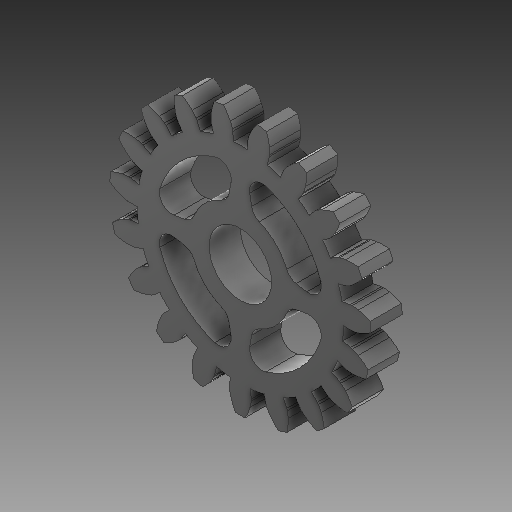
# Autodesk Inventor part: 歯車m2.z19
Saved by Autodesk Inventor 2020 (Build 240168000, 168)
## iProperties
Created: 2019-07-07
Part Number: 歯車m2.z19
Material: アセタール樹脂、黒
Document SubType Name: Modeling
Designer: 雪村
Density: 1.425 g/cm^3
Appearance: 滑らか - 黒
Mass: 5.2471 g
Surface Area: 35.7031 cm^2
Volume: 3.68217 cm^3
Description: ジュラコン 5t
Author: 雪村
Autodesk Inventor part; units mm, degrees
ref_plane "YZ Plane" through (0, 0, 0) normal (1, 0, 0) x (0, 1, 0)
ref_plane "XZ Plane" through (0, 0, 0) normal (0, 1, 0) x (-1, 0, 0)
ref_plane "XY Plane" through (0, 0, 0) normal (0, 0, 1) x (1, 0, 0)
sketch "スケッチ1" plane through (0, 0, 0) normal (0, 0, 1) x (1, 0, 0)
  arc A0 (20.2426, 88.5604) -> (20.1852, 88.263) centre (22.0204, 88.0631) ccw
  arc A1 (20.595, 89.4907) -> (20.2426, 88.5604) centre (25.1554, 87.231) ccw
  arc A2 (21.6786, 91.1755) -> (20.595, 89.4907) centre (28.5313, 85.5773) ccw
  arc A3 (14.2935, 87.9903) -> (14.3357, 87.6904) centre (16.1364, 88.0972) ccw
  arc A4 (14.3247, 88.9847) -> (14.2935, 87.9903) centre (19.3717, 88.3282) ccw
  arc A5 (14.8026, 90.93) -> (14.3247, 88.9847) centre (23.1017, 87.8602) ccw
  arc A6 (8.8518, 85.5195) -> (8.9892, 85.2495) centre (10.5602, 86.2189) ccw
  arc A7 (8.5585, 86.4701) -> (8.8518, 85.5195) centre (13.5452, 87.4879) ccw
  arc A8 (8.3788, 88.4651) -> (8.5585, 86.4701) centre (17.225, 88.2564) ccw
  arc A9 (4.5072, 81.4156) -> (4.7248, 81.2048) centre (5.8959, 82.6319) ccw
  arc A10 (3.9212, 82.2195) -> (4.5072, 81.4156) centre (8.3072, 84.8013) ccw
  arc A11 (3.1034, 84.0481) -> (3.9212, 82.2195) centre (11.5381, 86.723) ccw
  arc A12 (1.7306, 76.1234) -> (2.0048, 75.9947) centre (2.6491, 77.7247) ccw
  arc A13 (0.9153, 76.6934) -> (1.7306, 76.1234) centre (4.2253, 80.5595) ccw
  arc A14 (-0.4519, 78.1574) -> (0.9153, 76.6934) centre (6.6572, 83.4261) ccw
  arc A15 (0.8228, 70.2163) -> (1.124, 70.1837) centre (1.1716, 72.0291) ccw
  arc A16 (-0.1334, 70.4908) -> (0.8228, 70.2163) centre (1.742, 75.2221) ccw
  arc A17 (-1.9019, 71.4315) -> (-0.1334, 70.4908) centre (3.1113, 78.7231) ccw
  arc A18 (1.8822, 64.3346) -> (2.1776, 64.4015) centre (1.6235, 66.1624) ccw
  arc A19 (0.8887, 64.2837) -> (1.8822, 64.3346) centre (1.1262, 69.3676) ccw
  arc A20 (-1.0894, 64.5992) -> (0.8887, 64.2837) centre (1.2845, 73.1235) ccw
  arc A21 (4.794, 59.1156) -> (5.0517, 59.2748) centre (3.9558, 60.7604) ccw
  arc A22 (3.8708, 58.7448) -> (4.794, 59.1156) centre (2.4447, 63.6304) ccw
  arc A23 (1.8975, 58.401) -> (3.8708, 58.7448) centre (1.375, 67.2342) ccw
  arc A24 (9.2427, 55.1248) -> (9.4347, 55.359) centre (7.9158, 56.4083) ccw
  arc A25 (8.4899, 54.4743) -> (9.2427, 55.1248) centre (5.5547, 58.6321) ccw
  arc A26 (6.7351, 53.5084) -> (8.4899, 54.4743) centre (3.3728, 61.6933) ccw
  arc A27 (14.7461, 52.7947) -> (14.8516, 53.0786) centre (13.0744, 53.5778) ccw
  arc A28 (14.2453, 51.9351) -> (14.7461, 52.7947) centre (10.1191, 54.9145) ccw
  arc A29 (12.8992, 50.4516) -> (14.2453, 51.9351) centre (7.0614, 57.1014) ccw
  arc A30 (20.7079, 52.3778) -> (20.7155, 52.6806) centre (18.8725, 52.5757) ccw
  arc A31 (20.5134, 51.4021) -> (20.7079, 52.3778) centre (15.6433, 52.8804) ccw
  arc A32 (19.7219, 49.562) -> (20.5134, 51.4021) centre (12.0412, 53.9559) ccw
  arc A33 (26.482, 53.9192) -> (26.391, 54.2081) centre (24.6818, 53.5105) ccw
  arc A34 (26.6148, 52.9333) -> (26.482, 53.9192) centre (21.5286, 52.7502) ccw
  arc A35 (26.4637, 50.9359) -> (26.6148, 52.9333) centre (17.7725, 52.5978) ccw
  arc A36 (31.4428, 57.2521) -> (31.2629, 57.4958) centre (29.8729, 56.281) ccw
  arc A37 (31.8885, 56.3627) -> (31.4428, 57.2521) centre (27.1374, 54.538) ccw
  arc A38 (32.3942, 54.4244) -> (31.8885, 56.3627) centre (23.6343, 53.1743) ccw
  arc A39 (35.0526, 62.0151) -> (34.8033, 62.1871) centre (33.8831, 60.5868) ccw
  arc A40 (35.763, 61.3186) -> (35.0526, 62.0151) centre (31.8618, 58.0501) ccw
  arc A41 (36.8706, 59.6496) -> (35.763, 61.3186) centre (28.9912, 55.6228) ccw
  arc A42 (36.9203, 67.6921) -> (36.6286, 67.7739) centre (36.2779, 65.9615) ccw
  arc A43 (37.8183, 67.2641) -> (36.9203, 67.6921) centre (35.1898, 62.9059) ccw
  arc A44 (39.4078, 66.0451) -> (37.8183, 67.2641) centre (33.2629, 59.6781) ccw
  arc A45 (36.8435, 73.668) -> (36.541, 73.6506) centre (36.7978, 71.8225) ccw
  arc A46 (37.8318, 73.5547) -> (36.8435, 73.668) centre (36.7608, 68.5792) ccw
  arc A47 (39.731, 72.9179) -> (37.8318, 73.5547) centre (35.9864, 64.9006) ccw
  arc A48 (34.8304, 79.2951) -> (34.55, 79.1805) centre (35.3864, 77.5348) ccw
  arc A49 (35.802, 79.5089) -> (34.8304, 79.2951) centre (36.4045, 74.4552) ccw
  arc A50 (37.8051, 79.5233) -> (35.802, 79.5089) centre (36.8665, 70.7245) ccw
  arc A51 (31.0993, 83.9638) -> (30.8713, 83.7643) centre (32.1968, 82.4793) ccw
  arc A52 (31.9488, 84.4814) -> (31.0993, 83.9638) centre (34.1597, 79.8972) ccw
  arc A53 (33.8387, 85.1454) -> (31.9488, 84.4814) centre (35.808, 76.5186) ccw
  arc A54 (26.0545, 87.1679) -> (25.9036, 86.9052) centre (27.5744, 86.1203) ccw
  arc A55 (26.6899, 87.9334) -> (26.0545, 87.1679) centre (30.2694, 84.3154) ccw
  arc A56 (28.2618, 89.175) -> (26.6899, 87.9334) centre (32.9254, 81.6551) ccw
  arc A57 (17.7671, 88.263) -> (17.7097, 88.5604) centre (15.9319, 88.0631) ccw
  arc A58 (17.7097, 88.5604) -> (17.3572, 89.4907) centre (12.7969, 87.231) ccw
  arc A59 (17.3572, 89.4907) -> (16.2737, 91.1755) centre (9.421, 85.5773) ccw
  arc A60 (12.0487, 86.9052) -> (11.8978, 87.1679) centre (10.3778, 86.1203) ccw
  arc A61 (11.8978, 87.1679) -> (11.2624, 87.9334) centre (7.6829, 84.3154) ccw
  arc A62 (11.2624, 87.9334) -> (9.6905, 89.175) centre (5.0268, 81.6551) ccw
  arc A63 (7.081, 83.7643) -> (6.853, 83.9638) centre (5.7555, 82.4793) ccw
  arc A64 (6.853, 83.9638) -> (6.0034, 84.4814) centre (3.7926, 79.8972) ccw
  arc A65 (6.0034, 84.4814) -> (4.1136, 85.1454) centre (2.1443, 76.5186) ccw
  arc A66 (3.4023, 79.1805) -> (3.1219, 79.2951) centre (2.5659, 77.5348) ccw
  arc A67 (3.1219, 79.2951) -> (2.1503, 79.5089) centre (1.5477, 74.4552) ccw
  arc A68 (2.1503, 79.5089) -> (0.1472, 79.5233) centre (1.0857, 70.7245) ccw
  arc A69 (1.4112, 73.6506) -> (1.1088, 73.668) centre (1.1545, 71.8225) ccw
  arc A70 (1.1088, 73.668) -> (0.1205, 73.5547) centre (1.1915, 68.5792) ccw
  arc A71 (0.1205, 73.5547) -> (-1.7787, 72.9179) centre (1.9659, 64.9006) ccw
  arc A72 (1.3236, 67.7739) -> (1.032, 67.6921) centre (1.6744, 65.9615) ccw
  arc A73 (1.032, 67.6921) -> (0.134, 67.2641) centre (2.7625, 62.9059) ccw
  arc A74 (0.134, 67.2641) -> (-1.4556, 66.0451) centre (4.6894, 59.6781) ccw
  arc A75 (3.149, 62.1871) -> (2.8997, 62.0151) centre (4.0692, 60.5868) ccw
  arc A76 (2.8997, 62.0151) -> (2.1893, 61.3186) centre (6.0905, 58.0501) ccw
  arc A77 (2.1893, 61.3186) -> (1.0817, 59.6496) centre (8.961, 55.6228) ccw
  arc A78 (6.6894, 57.4958) -> (6.5095, 57.2521) centre (8.0794, 56.281) ccw
  arc A79 (6.5095, 57.2521) -> (6.0637, 56.3627) centre (10.8149, 54.538) ccw
  arc A80 (6.0637, 56.3627) -> (5.5581, 54.4244) centre (14.318, 53.1743) ccw
  arc A81 (11.5613, 54.2081) -> (11.4702, 53.9192) centre (13.2705, 53.5105) ccw
  arc A82 (11.4702, 53.9192) -> (11.3374, 52.9333) centre (16.4236, 52.7502) ccw
  arc A83 (11.3374, 52.9333) -> (11.4886, 50.9359) centre (20.1797, 52.5978) ccw
  arc A84 (17.2367, 52.6806) -> (17.2444, 52.3778) centre (19.0798, 52.5757) ccw
  arc A85 (17.2444, 52.3778) -> (17.4389, 51.4021) centre (22.309, 52.8804) ccw
  arc A86 (17.4389, 51.4021) -> (18.2304, 49.562) centre (25.9111, 53.9559) ccw
  arc A87 (23.1006, 53.0786) -> (23.2062, 52.7947) centre (24.8779, 53.5778) ccw
  arc A88 (23.2062, 52.7947) -> (23.707, 51.9351) centre (27.8332, 54.9145) ccw
  arc A89 (23.707, 51.9351) -> (25.0531, 50.4516) centre (30.8909, 57.1014) ccw
  arc A90 (28.5176, 55.359) -> (28.7096, 55.1248) centre (30.0364, 56.4083) ccw
  arc A91 (28.7096, 55.1248) -> (29.4624, 54.4743) centre (32.3976, 58.6321) ccw
  arc A92 (29.4624, 54.4743) -> (31.2172, 53.5084) centre (34.5795, 61.6933) ccw
  arc A93 (32.9006, 59.2748) -> (33.1583, 59.1156) centre (33.9964, 60.7604) ccw
  arc A94 (33.1583, 59.1156) -> (34.0814, 58.7448) centre (35.5076, 63.6304) ccw
  arc A95 (34.0814, 58.7448) -> (36.0548, 58.401) centre (36.5773, 67.2342) ccw
  arc A96 (35.7746, 64.4015) -> (36.0701, 64.3346) centre (36.3288, 66.1624) ccw
  arc A97 (36.0701, 64.3346) -> (37.0636, 64.2837) centre (36.8261, 69.3676) ccw
  arc A98 (37.0636, 64.2837) -> (39.0417, 64.5992) centre (36.6678, 73.1235) ccw
  arc A99 (36.8283, 70.1837) -> (37.1295, 70.2163) centre (36.7806, 72.0291) ccw
  arc A100 (37.1295, 70.2163) -> (38.0857, 70.4908) centre (36.2103, 75.2221) ccw
  arc A101 (38.0857, 70.4908) -> (39.8542, 71.4315) centre (34.841, 78.7231) ccw
  arc A102 (35.9474, 75.9947) -> (36.2217, 76.1234) centre (35.3031, 77.7247) ccw
  arc A103 (36.2217, 76.1234) -> (37.037, 76.6934) centre (33.727, 80.5595) ccw
  arc A104 (37.037, 76.6934) -> (38.4042, 78.1574) centre (31.2951, 83.4261) ccw
  arc A105 (33.2275, 81.2048) -> (33.4451, 81.4156) centre (32.0563, 82.6319) ccw
  arc A106 (33.4451, 81.4156) -> (34.0311, 82.2195) centre (29.6451, 84.8013) ccw
  arc A107 (34.0311, 82.2195) -> (34.8489, 84.0481) centre (26.4142, 86.723) ccw
  arc A108 (28.9631, 85.2495) -> (29.1005, 85.5195) centre (27.3921, 86.2189) ccw
  arc A109 (29.1005, 85.5195) -> (29.3938, 86.4701) centre (24.4071, 87.4879) ccw
  arc A110 (29.3938, 86.4701) -> (29.5735, 88.4651) centre (20.7273, 88.2564) ccw
  arc A111 (23.6165, 87.6904) -> (23.6588, 87.9903) centre (21.8159, 88.0972) ccw
  arc A112 (23.6588, 87.9903) -> (23.6275, 88.9847) centre (18.5806, 88.3282) ccw
  arc A113 (23.6275, 88.9847) -> (23.1497, 90.93) centre (14.8506, 87.8602) ccw
  arc A114 (20.0935, 86.9119) -> (17.8588, 86.9119) centre (18.9761, 70.4498) ccw
  arc A115 (14.6877, 86.3828) -> (12.5741, 85.6572) centre (18.9761, 70.4498) ccw
  arc A116 (9.7466, 84.127) -> (7.9832, 82.7545) centre (18.9761, 70.4498) ccw
  arc A117 (5.8057, 80.3891) -> (4.5835, 78.5183) centre (18.9761, 70.4498) ccw
  arc A118 (3.292, 75.5742) -> (2.7435, 73.4079) centre (18.9761, 70.4498) ccw
  arc A119 (2.478, 70.2039) -> (2.6625, 67.9769) centre (18.9761, 70.4498) ccw
  arc A120 (3.4517, 64.8603) -> (4.3494, 62.8138) centre (18.9761, 70.4498) ccw
  arc A121 (6.1078, 60.1224) -> (7.6213, 58.4783) centre (18.9761, 70.4498) ccw
  arc A122 (10.1584, 56.5036) -> (12.1237, 55.44) centre (18.9761, 70.4498) ccw
  arc A123 (15.1645, 54.3961) -> (17.3687, 54.0283) centre (18.9761, 70.4498) ccw
  arc A124 (20.5836, 54.0283) -> (22.7878, 54.3961) centre (18.9761, 70.4498) ccw
  arc A125 (25.8286, 55.44) -> (27.7939, 56.5036) centre (18.9761, 70.4498) ccw
  arc A126 (30.331, 58.4783) -> (31.8445, 60.1224) centre (18.9761, 70.4498) ccw
  arc A127 (33.6029, 62.8138) -> (34.5005, 64.8603) centre (18.9761, 70.4498) ccw
  arc A128 (35.2898, 67.9769) -> (35.4743, 70.2039) centre (18.9761, 70.4498) ccw
  arc A129 (35.2088, 73.4079) -> (34.6602, 75.5742) centre (18.9761, 70.4498) ccw
  arc A130 (33.3688, 78.5183) -> (32.1466, 80.3891) centre (18.9761, 70.4498) ccw
  arc A131 (29.9691, 82.7545) -> (28.2057, 84.127) centre (18.9761, 70.4498) ccw
  arc A132 (25.3782, 85.6572) -> (23.2646, 86.3828) centre (18.9761, 70.4498) ccw
  arc A133 (16.2737, 91.1755) -> (14.8026, 90.93) centre (18.9761, 70.4498) ccw
  arc A134 (9.6905, 89.175) -> (8.3788, 88.4651) centre (18.9761, 70.4498) ccw
  arc A135 (4.1136, 85.1454) -> (3.1034, 84.0481) centre (18.9761, 70.4498) ccw
  arc A136 (0.1472, 79.5233) -> (-0.4519, 78.1574) centre (18.9761, 70.4498) ccw
  arc A137 (-1.7787, 72.9179) -> (-1.9019, 71.4315) centre (18.9761, 70.4498) ccw
  arc A138 (-1.4556, 66.0451) -> (-1.0894, 64.5992) centre (18.9761, 70.4498) ccw
  arc A139 (1.0817, 59.6496) -> (1.8975, 58.401) centre (18.9761, 70.4498) ccw
  arc A140 (5.5581, 54.4244) -> (6.7351, 53.5084) centre (18.9761, 70.4498) ccw
  arc A141 (11.4886, 50.9359) -> (12.8992, 50.4516) centre (18.9761, 70.4498) ccw
  arc A142 (18.2304, 49.562) -> (19.7219, 49.562) centre (18.9761, 70.4498) ccw
  arc A143 (25.0531, 50.4516) -> (26.4637, 50.9359) centre (18.9761, 70.4498) ccw
  arc A144 (31.2172, 53.5084) -> (32.3942, 54.4244) centre (18.9761, 70.4498) ccw
  arc A145 (36.0548, 58.401) -> (36.8706, 59.6496) centre (18.9761, 70.4498) ccw
  arc A146 (39.0417, 64.5992) -> (39.4078, 66.0451) centre (18.9761, 70.4498) ccw
  arc A147 (39.8542, 71.4315) -> (39.731, 72.9179) centre (18.9761, 70.4498) ccw
  arc A148 (38.4042, 78.1574) -> (37.8051, 79.5233) centre (18.9761, 70.4498) ccw
  arc A149 (34.8489, 84.0481) -> (33.8387, 85.1454) centre (18.9761, 70.4498) ccw
  arc A150 (29.5735, 88.4651) -> (28.2618, 89.175) centre (18.9761, 70.4498) ccw
  arc A151 (23.1497, 90.93) -> (21.6786, 91.1755) centre (18.9761, 70.4498) ccw
  line L0 (20.0935, 86.9119) -> (20.1852, 88.263)
  line L1 (14.6877, 86.3828) -> (14.3357, 87.6904)
  line L2 (9.7466, 84.127) -> (8.9892, 85.2495)
  line L3 (5.8057, 80.3891) -> (4.7248, 81.2048)
  line L4 (3.292, 75.5742) -> (2.0048, 75.9947)
  line L5 (2.478, 70.2039) -> (1.124, 70.1837)
  line L6 (3.4517, 64.8603) -> (2.1776, 64.4015)
  line L7 (6.1078, 60.1224) -> (5.0517, 59.2748)
  line L8 (10.1584, 56.5036) -> (9.4347, 55.359)
  line L9 (15.1645, 54.3961) -> (14.8516, 53.0786)
  line L10 (20.5836, 54.0283) -> (20.7155, 52.6806)
  line L11 (25.8286, 55.44) -> (26.391, 54.2081)
  line L12 (30.331, 58.4783) -> (31.2629, 57.4958)
  line L13 (33.6029, 62.8138) -> (34.8033, 62.1871)
  line L14 (35.2898, 67.9769) -> (36.6286, 67.7739)
  line L15 (35.2088, 73.4079) -> (36.541, 73.6506)
  line L16 (33.3688, 78.5183) -> (34.55, 79.1805)
  line L17 (29.9691, 82.7545) -> (30.8713, 83.7643)
  line L18 (25.3782, 85.6572) -> (25.9036, 86.9052)
  line L19 (17.8588, 86.9119) -> (17.7671, 88.263)
  line L20 (12.5741, 85.6572) -> (12.0487, 86.9052)
  line L21 (7.9832, 82.7545) -> (7.081, 83.7643)
  line L22 (4.5835, 78.5183) -> (3.4023, 79.1805)
  line L23 (2.7435, 73.4079) -> (1.4112, 73.6506)
  line L24 (2.6625, 67.9769) -> (1.3236, 67.7739)
  line L25 (4.3494, 62.8138) -> (3.149, 62.1871)
  line L26 (7.6213, 58.4783) -> (6.6894, 57.4958)
  line L27 (12.1237, 55.44) -> (11.5613, 54.2081)
  line L28 (17.3687, 54.0283) -> (17.2367, 52.6806)
  line L29 (22.7878, 54.3961) -> (23.1006, 53.0786)
  line L30 (27.7939, 56.5036) -> (28.5176, 55.359)
  line L31 (31.8445, 60.1224) -> (32.9006, 59.2748)
  line L32 (34.5005, 64.8603) -> (35.7746, 64.4015)
  line L33 (35.4743, 70.2039) -> (36.8283, 70.1837)
  line L34 (34.6602, 75.5742) -> (35.9474, 75.9947)
  line L35 (32.1466, 80.3891) -> (33.2275, 81.2048)
  line L36 (28.2057, 84.127) -> (28.9631, 85.2495)
  line L37 (23.2646, 86.3828) -> (23.6165, 87.6904)
  line L38 (-3.925, 70.4498) -> (41.8772, 70.4498)
  line L39 (18.9761, 47.5487) -> (18.9761, 93.3509)
  line L40 (59.8772, 91.3509) -> (129.8772, 91.3509)
  line L41 (59.8772, 83.3509) -> (129.8772, 83.3509)
  line L42 (59.8772, 75.3509) -> (129.8772, 75.3509)
  line L43 (59.8772, 67.3509) -> (129.8772, 67.3509)
  line L44 (59.8772, 59.3509) -> (129.8772, 59.3509)
  line L45 (59.8772, 51.3509) -> (129.8772, 51.3509)
  line L46 (59.8772, 43.3509) -> (129.8772, 43.3509)
  line L47 (59.8772, 35.3509) -> (129.8772, 35.3509)
  line L48 (59.8772, 27.3509) -> (129.8772, 27.3509)
  line L49 (59.8772, 19.3509) -> (129.8772, 19.3509)
  line L50 (59.8772, 11.3509) -> (129.8772, 11.3509)
  line L51 (59.8772, 3.3509) -> (129.8772, 3.3509)
  line L52 (59.8772, -4.6491) -> (129.8772, -4.6491)
  line L53 (59.8772, 91.3509) -> (59.8772, -4.6491)
  line L54 (129.8772, 91.3509) -> (129.8772, -4.6491)
  line L55 (94.8772, 83.3509) -> (94.8772, -4.6491)
  point P0 (0, 0)
  point P1 (0, 0)
  point P2 (65.8772, 85.3509)
  point P3 (68.3772, 77.3509)
  point P4 (68.3772, 69.3509)
  point P5 (65.8772, 61.3509)
  point P6 (68.3772, 53.3509)
  point P7 (63.3772, 45.3509)
  point P8 (65.8772, 37.3509)
  point P9 (65.8772, 29.3509)
  point P10 (65.8772, 21.3509)
  point P11 (68.3772, 13.3509)
  point P12 (68.3772, 5.3509)
  point P13 (65.8772, -2.6491)
  point P14 (95.8772, 77.3509)
  point P15 (110.8772, 69.3509)
  point P16 (112.1272, 61.3509)
  point P17 (108.3772, 53.3509)
  point P18 (110.8772, 45.3509)
  point P19 (104.6272, 37.3509)
  point P20 (104.6272, 29.3509)
  point P21 (110.8772, 21.3509)
  point P22 (105.8772, 13.3509)
  point P23 (19.9761, 106.8509)
  point P24 (19.9761, 100.8509)
  point P25 (36.1636, 106.8509)
  point P26 (39.3511, 100.8509)
  constraints: 228 point on circle, 114 centre point, 108 end point, 2 horizontal alignment, 2 midpoint, 165 other
extrude "押し出し1" add sketch "スケッチ1" along normal blind 5 contours A1 A2 A151 A113 A112 A111 L37 A132 L18 A54 A55 A56 A150 A110 A109 A108 L36 A131 L17 A51 A52 A53 A149 A107 A106 A105 L35 A130 L16 A48 A49 A50 A148 A104 A103 A102 L34 A129 L15 A45 A46 A47 A147 A101 A100 L38 L39 A114 L0 A0 | L39 L38 A16 A17 A137 A71 A70 A69 L23 A118 L4 A12 A13 A14 A136 A68 A67 A66 L22 A117 L3 A9 A10 A11 A135 A65 A64 A63 L21 A116 L2 A6 A7 A8 A134 A62 A61 A60 L20 A115 L1 A3 A4 A5 A133 A59 A58 A57 L19 A114 | L39 A142 A86 A85 A84 L28 A123 L9 A27 A28 A29 A141 A83 A82 A81 L27 A122 L8 A24 A25 A26 A140 A80 A79 A78 L26 A121 L7 A21 A22 A23 A139 A77 A76 A75 L25 A120 L6 A18 A19 A20 A138 A74 A73 A72 L24 A119 L5 A15 A16 L38 | L38 A100 A99 L33 A128 L14 A42 A43 A44 A146 A98 A97 A96 L32 A127 L13 A39 A40 A41 A145 A95 A94 A93 L31 A126 L12 A36 A37 A38 A144 A92 A91 A90 L30 A125 L11 A33 A34 A35 A143 A89 A88 A87 L29 A124 L10 A30 A31 A32 A142 L39
sketch "スケッチ2" plane through (0, 0, 5) normal (0, 0, 1) x (1, 0, 0)
  arc A0 (6.5095, 57.2521) -> (6.0637, 56.3627) centre (10.8149, 54.538) ccw projected
  arc A1 (6.0637, 56.3627) -> (5.5581, 54.4244) centre (14.318, 53.1743) ccw projected
  arc A2 (5.5581, 54.4244) -> (6.7351, 53.5084) centre (18.9761, 70.4498) ccw projected
  arc A3 (6.7351, 53.5084) -> (8.4899, 54.4743) centre (3.3728, 61.6933) ccw projected
  arc A4 (8.4899, 54.4743) -> (9.2427, 55.1248) centre (5.5547, 58.6321) ccw projected
  arc A5 (9.2427, 55.1248) -> (9.4347, 55.359) centre (7.9158, 56.4083) ccw projected
  line L0 (9.4347, 55.359) -> (10.1584, 56.5036) projected
  arc A6 (10.1584, 56.5036) -> (12.1237, 55.44) centre (18.9761, 70.4498) ccw projected
  line L1 (12.1237, 55.44) -> (11.5613, 54.2081) projected
  arc A7 (11.5613, 54.2081) -> (11.4702, 53.9192) centre (13.2705, 53.5105) ccw projected
  arc A8 (11.4702, 53.9192) -> (11.3374, 52.9333) centre (16.4236, 52.7502) ccw projected
  arc A9 (11.3374, 52.9333) -> (11.4886, 50.9359) centre (20.1797, 52.5978) ccw projected
  arc A10 (11.4886, 50.9359) -> (12.8992, 50.4516) centre (18.9761, 70.4498) ccw projected
  arc A11 (12.8992, 50.4516) -> (14.2453, 51.9351) centre (7.0614, 57.1014) ccw projected
  arc A12 (14.2453, 51.9351) -> (14.7461, 52.7947) centre (10.1191, 54.9145) ccw projected
  arc A13 (14.7461, 52.7947) -> (14.8516, 53.0786) centre (13.0744, 53.5778) ccw projected
  line L2 (14.8516, 53.0786) -> (15.1645, 54.3961) projected
  arc A14 (15.1645, 54.3961) -> (17.3687, 54.0283) centre (18.9761, 70.4498) ccw projected
  line L3 (17.3687, 54.0283) -> (17.2367, 52.6806) projected
  arc A15 (17.2367, 52.6806) -> (17.2444, 52.3778) centre (19.0798, 52.5757) ccw projected
  arc A16 (17.2444, 52.3778) -> (17.4389, 51.4021) centre (22.309, 52.8804) ccw projected
  arc A17 (17.4389, 51.4021) -> (18.2304, 49.562) centre (25.9111, 53.9559) ccw projected
  arc A18 (18.2304, 49.562) -> (19.7219, 49.562) centre (18.9761, 70.4498) ccw projected
  arc A19 (19.7219, 49.562) -> (20.5134, 51.4021) centre (12.0412, 53.9559) ccw projected
  arc A20 (20.5134, 51.4021) -> (20.7079, 52.3778) centre (15.6433, 52.8804) ccw projected
  arc A21 (20.7079, 52.3778) -> (20.7155, 52.6806) centre (18.8725, 52.5757) ccw projected
  line L4 (20.7155, 52.6806) -> (20.5836, 54.0283) projected
  arc A22 (20.5836, 54.0283) -> (22.7878, 54.3961) centre (18.9761, 70.4498) ccw projected
  line L5 (22.7878, 54.3961) -> (23.1006, 53.0786) projected
  arc A23 (23.1006, 53.0786) -> (23.2062, 52.7947) centre (24.8779, 53.5778) ccw projected
  arc A24 (23.2062, 52.7947) -> (23.707, 51.9351) centre (27.8332, 54.9145) ccw projected
  arc A25 (23.707, 51.9351) -> (25.0531, 50.4516) centre (30.8909, 57.1014) ccw projected
  arc A26 (25.0531, 50.4516) -> (26.4637, 50.9359) centre (18.9761, 70.4498) ccw projected
  arc A27 (26.4637, 50.9359) -> (26.6148, 52.9333) centre (17.7725, 52.5978) ccw projected
  arc A28 (26.6148, 52.9333) -> (26.482, 53.9192) centre (21.5286, 52.7502) ccw projected
  arc A29 (26.482, 53.9192) -> (26.391, 54.2081) centre (24.6818, 53.5105) ccw projected
  line L6 (26.391, 54.2081) -> (25.8286, 55.44) projected
  arc A30 (25.8286, 55.44) -> (27.7939, 56.5036) centre (18.9761, 70.4498) ccw projected
  line L7 (27.7939, 56.5036) -> (28.5176, 55.359) projected
  arc A31 (28.5176, 55.359) -> (28.7096, 55.1248) centre (30.0364, 56.4083) ccw projected
  arc A32 (28.7096, 55.1248) -> (29.4624, 54.4743) centre (32.3976, 58.6321) ccw projected
  arc A33 (29.4624, 54.4743) -> (31.2172, 53.5084) centre (34.5795, 61.6933) ccw projected
  arc A34 (31.2172, 53.5084) -> (32.3942, 54.4244) centre (18.9761, 70.4498) ccw projected
  arc A35 (32.3942, 54.4244) -> (31.8885, 56.3627) centre (23.6343, 53.1743) ccw projected
  arc A36 (31.8885, 56.3627) -> (31.4428, 57.2521) centre (27.1374, 54.538) ccw projected
  arc A37 (31.4428, 57.2521) -> (31.2629, 57.4958) centre (29.8729, 56.281) ccw projected
  line L8 (31.2629, 57.4958) -> (30.331, 58.4783) projected
  arc A38 (30.331, 58.4783) -> (31.8445, 60.1224) centre (18.9761, 70.4498) ccw projected
  line L9 (31.8445, 60.1224) -> (32.9006, 59.2748) projected
  arc A39 (32.9006, 59.2748) -> (33.1583, 59.1156) centre (33.9964, 60.7604) ccw projected
  arc A40 (33.1583, 59.1156) -> (34.0814, 58.7448) centre (35.5076, 63.6304) ccw projected
  arc A41 (34.0814, 58.7448) -> (36.0548, 58.401) centre (36.5773, 67.2342) ccw projected
  arc A42 (36.0548, 58.401) -> (36.8706, 59.6496) centre (18.9761, 70.4498) ccw projected
  arc A43 (36.8706, 59.6496) -> (35.763, 61.3186) centre (28.9912, 55.6228) ccw projected
  arc A44 (35.763, 61.3186) -> (35.0526, 62.0151) centre (31.8618, 58.0501) ccw projected
  arc A45 (35.0526, 62.0151) -> (34.8033, 62.1871) centre (33.8831, 60.5868) ccw projected
  line L10 (34.8033, 62.1871) -> (33.6029, 62.8138) projected
  arc A46 (33.6029, 62.8138) -> (34.5005, 64.8603) centre (18.9761, 70.4498) ccw projected
  line L11 (34.5005, 64.8603) -> (35.7746, 64.4015) projected
  arc A47 (35.7746, 64.4015) -> (36.0701, 64.3346) centre (36.3288, 66.1624) ccw projected
  arc A48 (36.0701, 64.3346) -> (37.0636, 64.2837) centre (36.8261, 69.3676) ccw projected
  arc A49 (37.0636, 64.2837) -> (39.0417, 64.5992) centre (36.6678, 73.1235) ccw projected
  arc A50 (39.0417, 64.5992) -> (39.4078, 66.0451) centre (18.9761, 70.4498) ccw projected
  arc A51 (39.4078, 66.0451) -> (37.8183, 67.2641) centre (33.2629, 59.6781) ccw projected
  arc A52 (37.8183, 67.2641) -> (36.9203, 67.6921) centre (35.1898, 62.9059) ccw projected
  arc A53 (36.9203, 67.6921) -> (36.6286, 67.7739) centre (36.2779, 65.9615) ccw projected
  line L12 (36.6286, 67.7739) -> (35.2898, 67.9769) projected
  arc A54 (35.2898, 67.9769) -> (35.4743, 70.2039) centre (18.9761, 70.4498) ccw projected
  line L13 (35.4743, 70.2039) -> (36.8283, 70.1837) projected
  arc A55 (36.8283, 70.1837) -> (37.1295, 70.2163) centre (36.7806, 72.0291) ccw projected
  arc A56 (37.1295, 70.2163) -> (38.0857, 70.4908) centre (36.2103, 75.2221) ccw projected
  arc A57 (38.0857, 70.4908) -> (39.8542, 71.4315) centre (34.841, 78.7231) ccw projected
  arc A58 (39.8542, 71.4315) -> (39.731, 72.9179) centre (18.9761, 70.4498) ccw projected
  arc A59 (39.731, 72.9179) -> (37.8318, 73.5547) centre (35.9864, 64.9006) ccw projected
  arc A60 (37.8318, 73.5547) -> (36.8435, 73.668) centre (36.7608, 68.5792) ccw projected
  arc A61 (36.8435, 73.668) -> (36.541, 73.6506) centre (36.7978, 71.8225) ccw projected
  line L14 (36.541, 73.6506) -> (35.2088, 73.4079) projected
  arc A62 (35.2088, 73.4079) -> (34.6602, 75.5742) centre (18.9761, 70.4498) ccw projected
  line L15 (34.6602, 75.5742) -> (35.9474, 75.9947) projected
  arc A63 (35.9474, 75.9947) -> (36.2217, 76.1234) centre (35.3031, 77.7247) ccw projected
  arc A64 (36.2217, 76.1234) -> (37.037, 76.6934) centre (33.727, 80.5595) ccw projected
  arc A65 (37.037, 76.6934) -> (38.4042, 78.1574) centre (31.2951, 83.4261) ccw projected
  arc A66 (38.4042, 78.1574) -> (37.8051, 79.5233) centre (18.9761, 70.4498) ccw projected
  arc A67 (37.8051, 79.5233) -> (35.802, 79.5089) centre (36.8665, 70.7245) ccw projected
  arc A68 (35.802, 79.5089) -> (34.8304, 79.2951) centre (36.4045, 74.4552) ccw projected
  arc A69 (34.8304, 79.2951) -> (34.55, 79.1805) centre (35.3864, 77.5348) ccw projected
  line L16 (34.55, 79.1805) -> (33.3688, 78.5183) projected
  arc A70 (33.3688, 78.5183) -> (32.1466, 80.3891) centre (18.9761, 70.4498) ccw projected
  line L17 (32.1466, 80.3891) -> (33.2275, 81.2048) projected
  arc A71 (33.2275, 81.2048) -> (33.4451, 81.4156) centre (32.0563, 82.6319) ccw projected
  arc A72 (33.4451, 81.4156) -> (34.0311, 82.2195) centre (29.6451, 84.8013) ccw projected
  arc A73 (34.0311, 82.2195) -> (34.8489, 84.0481) centre (26.4142, 86.723) ccw projected
  arc A74 (34.8489, 84.0481) -> (33.8387, 85.1454) centre (18.9761, 70.4498) ccw projected
  arc A75 (33.8387, 85.1454) -> (31.9488, 84.4814) centre (35.808, 76.5186) ccw projected
  arc A76 (31.9488, 84.4814) -> (31.0993, 83.9638) centre (34.1597, 79.8972) ccw projected
  arc A77 (31.0993, 83.9638) -> (30.8713, 83.7643) centre (32.1968, 82.4793) ccw projected
  line L18 (30.8713, 83.7643) -> (29.9691, 82.7545) projected
  arc A78 (29.9691, 82.7545) -> (28.2057, 84.127) centre (18.9761, 70.4498) ccw projected
  line L19 (28.2057, 84.127) -> (28.9631, 85.2495) projected
  arc A79 (28.9631, 85.2495) -> (29.1005, 85.5195) centre (27.3921, 86.2189) ccw projected
  arc A80 (29.1005, 85.5195) -> (29.3938, 86.4701) centre (24.4071, 87.4879) ccw projected
  arc A81 (29.3938, 86.4701) -> (29.5735, 88.4651) centre (20.7273, 88.2564) ccw projected
  arc A82 (29.5735, 88.4651) -> (28.2618, 89.175) centre (18.9761, 70.4498) ccw projected
  arc A83 (28.2618, 89.175) -> (26.6899, 87.9334) centre (32.9254, 81.6551) ccw projected
  arc A84 (26.6899, 87.9334) -> (26.0545, 87.1679) centre (30.2694, 84.3154) ccw projected
  arc A85 (26.0545, 87.1679) -> (25.9036, 86.9052) centre (27.5744, 86.1203) ccw projected
  line L20 (25.9036, 86.9052) -> (25.3782, 85.6572) projected
  arc A86 (25.3782, 85.6572) -> (23.2646, 86.3828) centre (18.9761, 70.4498) ccw projected
  line L21 (23.2646, 86.3828) -> (23.6165, 87.6904) projected
  arc A87 (23.6165, 87.6904) -> (23.6588, 87.9903) centre (21.8159, 88.0972) ccw projected
  arc A88 (23.6588, 87.9903) -> (23.6275, 88.9847) centre (18.5806, 88.3282) ccw projected
  arc A89 (23.6275, 88.9847) -> (23.1497, 90.93) centre (14.8506, 87.8602) ccw projected
  arc A90 (23.1497, 90.93) -> (21.6786, 91.1755) centre (18.9761, 70.4498) ccw projected
  arc A91 (21.6786, 91.1755) -> (20.595, 89.4907) centre (28.5313, 85.5773) ccw projected
  arc A92 (20.595, 89.4907) -> (20.2426, 88.5604) centre (25.1554, 87.231) ccw projected
  arc A93 (20.2426, 88.5604) -> (20.1852, 88.263) centre (22.0204, 88.0631) ccw projected
  line L22 (20.1852, 88.263) -> (20.0935, 86.9119) projected
  arc A94 (20.0935, 86.9119) -> (17.8588, 86.9119) centre (18.9761, 70.4498) ccw projected
  line L23 (17.8588, 86.9119) -> (17.7671, 88.263) projected
  arc A95 (17.7671, 88.263) -> (17.7097, 88.5604) centre (15.9319, 88.0631) ccw projected
  arc A96 (17.7097, 88.5604) -> (17.3572, 89.4907) centre (12.7969, 87.231) ccw projected
  arc A97 (17.3572, 89.4907) -> (16.2737, 91.1755) centre (9.421, 85.5773) ccw projected
  arc A98 (16.2737, 91.1755) -> (14.8026, 90.93) centre (18.9761, 70.4498) ccw projected
  arc A99 (14.8026, 90.93) -> (14.3247, 88.9847) centre (23.1017, 87.8602) ccw projected
  arc A100 (14.3247, 88.9847) -> (14.2935, 87.9903) centre (19.3717, 88.3282) ccw projected
  arc A101 (14.2935, 87.9903) -> (14.3357, 87.6904) centre (16.1364, 88.0972) ccw projected
  line L24 (14.3357, 87.6904) -> (14.6877, 86.3828) projected
  arc A102 (14.6877, 86.3828) -> (12.5741, 85.6572) centre (18.9761, 70.4498) ccw projected
  line L25 (12.5741, 85.6572) -> (12.0487, 86.9052) projected
  arc A103 (12.0487, 86.9052) -> (11.8978, 87.1679) centre (10.3778, 86.1203) ccw projected
  arc A104 (11.8978, 87.1679) -> (11.2624, 87.9334) centre (7.6829, 84.3154) ccw projected
  arc A105 (11.2624, 87.9334) -> (9.6905, 89.175) centre (5.0268, 81.6551) ccw projected
  arc A106 (9.6905, 89.175) -> (8.3788, 88.4651) centre (18.9761, 70.4498) ccw projected
  arc A107 (8.3788, 88.4651) -> (8.5585, 86.4701) centre (17.225, 88.2564) ccw projected
  arc A108 (8.5585, 86.4701) -> (8.8518, 85.5195) centre (13.5452, 87.4879) ccw projected
  arc A109 (8.8518, 85.5195) -> (8.9892, 85.2495) centre (10.5602, 86.2189) ccw projected
  line L26 (8.9892, 85.2495) -> (9.7466, 84.127) projected
  arc A110 (9.7466, 84.127) -> (7.9832, 82.7545) centre (18.9761, 70.4498) ccw projected
  line L27 (7.9832, 82.7545) -> (7.081, 83.7643) projected
  arc A111 (7.081, 83.7643) -> (6.853, 83.9638) centre (5.7555, 82.4793) ccw projected
  arc A112 (6.853, 83.9638) -> (6.0034, 84.4814) centre (3.7926, 79.8972) ccw projected
  arc A113 (6.0034, 84.4814) -> (4.1136, 85.1454) centre (2.1443, 76.5186) ccw projected
  arc A114 (4.1136, 85.1454) -> (3.1034, 84.0481) centre (18.9761, 70.4498) ccw projected
  arc A115 (3.1034, 84.0481) -> (3.9212, 82.2195) centre (11.5381, 86.723) ccw projected
  arc A116 (3.9212, 82.2195) -> (4.5072, 81.4156) centre (8.3072, 84.8013) ccw projected
  arc A117 (4.5072, 81.4156) -> (4.7248, 81.2048) centre (5.8959, 82.6319) ccw projected
  line L28 (4.7248, 81.2048) -> (5.8057, 80.3891) projected
  arc A118 (5.8057, 80.3891) -> (4.5835, 78.5183) centre (18.9761, 70.4498) ccw projected
  line L29 (4.5835, 78.5183) -> (3.4023, 79.1805) projected
  arc A119 (3.4023, 79.1805) -> (3.1219, 79.2951) centre (2.5659, 77.5348) ccw projected
  arc A120 (3.1219, 79.2951) -> (2.1503, 79.5089) centre (1.5477, 74.4552) ccw projected
  arc A121 (2.1503, 79.5089) -> (0.1472, 79.5233) centre (1.0857, 70.7245) ccw projected
  arc A122 (0.1472, 79.5233) -> (-0.4519, 78.1574) centre (18.9761, 70.4498) ccw projected
  arc A123 (-0.4519, 78.1574) -> (0.9153, 76.6934) centre (6.6572, 83.4261) ccw projected
  arc A124 (0.9153, 76.6934) -> (1.7306, 76.1234) centre (4.2253, 80.5595) ccw projected
  arc A125 (1.7306, 76.1234) -> (2.0048, 75.9947) centre (2.6491, 77.7247) ccw projected
  line L30 (2.0048, 75.9947) -> (3.292, 75.5742) projected
  arc A126 (3.292, 75.5742) -> (2.7435, 73.4079) centre (18.9761, 70.4498) ccw projected
  line L31 (2.7435, 73.4079) -> (1.4112, 73.6506) projected
  arc A127 (1.4112, 73.6506) -> (1.1088, 73.668) centre (1.1545, 71.8225) ccw projected
  arc A128 (1.1088, 73.668) -> (0.1205, 73.5547) centre (1.1915, 68.5792) ccw projected
  arc A129 (0.1205, 73.5547) -> (-1.7787, 72.9179) centre (1.9659, 64.9006) ccw projected
  arc A130 (-1.7787, 72.9179) -> (-1.9019, 71.4315) centre (18.9761, 70.4498) ccw projected
  arc A131 (-1.9019, 71.4315) -> (-0.1334, 70.4908) centre (3.1113, 78.7231) ccw projected
  arc A132 (-0.1334, 70.4908) -> (0.8228, 70.2163) centre (1.742, 75.2221) ccw projected
  arc A133 (0.8228, 70.2163) -> (1.124, 70.1837) centre (1.1716, 72.0291) ccw projected
  line L32 (1.124, 70.1837) -> (2.478, 70.2039) projected
  arc A134 (2.478, 70.2039) -> (2.6625, 67.9769) centre (18.9761, 70.4498) ccw projected
  line L33 (2.6625, 67.9769) -> (1.3236, 67.7739) projected
  arc A135 (1.3236, 67.7739) -> (1.032, 67.6921) centre (1.6744, 65.9615) ccw projected
  arc A136 (1.032, 67.6921) -> (0.134, 67.2641) centre (2.7625, 62.9059) ccw projected
  arc A137 (0.134, 67.2641) -> (-1.4556, 66.0451) centre (4.6894, 59.6781) ccw projected
  arc A138 (-1.4556, 66.0451) -> (-1.0894, 64.5992) centre (18.9761, 70.4498) ccw projected
  arc A139 (-1.0894, 64.5992) -> (0.8887, 64.2837) centre (1.2845, 73.1235) ccw projected
  arc A140 (0.8887, 64.2837) -> (1.8822, 64.3346) centre (1.1262, 69.3676) ccw projected
  arc A141 (1.8822, 64.3346) -> (2.1776, 64.4015) centre (1.6235, 66.1624) ccw projected
  line L34 (2.1776, 64.4015) -> (3.4517, 64.8603) projected
  arc A142 (3.4517, 64.8603) -> (4.3494, 62.8138) centre (18.9761, 70.4498) ccw projected
  line L35 (4.3494, 62.8138) -> (3.149, 62.1871) projected
  arc A143 (3.149, 62.1871) -> (2.8997, 62.0151) centre (4.0692, 60.5868) ccw projected
  arc A144 (2.8997, 62.0151) -> (2.1893, 61.3186) centre (6.0905, 58.0501) ccw projected
  arc A145 (2.1893, 61.3186) -> (1.0817, 59.6496) centre (8.961, 55.6228) ccw projected
  arc A146 (1.0817, 59.6496) -> (1.8975, 58.401) centre (18.9761, 70.4498) ccw projected
  arc A147 (1.8975, 58.401) -> (3.8708, 58.7448) centre (1.375, 67.2342) ccw projected
  arc A148 (3.8708, 58.7448) -> (4.794, 59.1156) centre (2.4447, 63.6304) ccw projected
  arc A149 (4.794, 59.1156) -> (5.0517, 59.2748) centre (3.9558, 60.7604) ccw projected
  line L36 (5.0517, 59.2748) -> (6.1078, 60.1224) projected
  arc A150 (6.1078, 60.1224) -> (7.6213, 58.4783) centre (18.9761, 70.4498) ccw projected
  line L37 (7.6213, 58.4783) -> (6.6894, 57.4958) projected
  arc A151 (6.6894, 57.4958) -> (6.5095, 57.2521) centre (8.0794, 56.281) ccw projected
  circle A152 centre (18.9761, 70.4498) radius 5
  point P0 (0, 0)
  dimension "d2" = 10
  constraints: 1 centre point, 1 coincident
  measures "d2" diameter of A152
extrude "押し出し2" cut sketch "スケッチ2" against normal through all contours A152
sketch "スケッチ3" plane through (0, 0, 5) normal (0, 0, 1) x (1, 0, 0)
  circle A0 centre (18.9761, 70.4498) radius 5 projected
  circle A1 centre (18.9761, 70.4498) radius 16.5
  circle A2 centre (18.9761, 70.4498) radius 13.5
  circle A3 centre (18.9761, 70.4498) radius 8
  point P0 (0, 0)
  point P1 (14.6877, 86.3828)
  dimension "d5" = 3
  dimension "d6" = 3
  constraints: 2 centre point, 1 coincident, 3 other
  measures "d6" radial gap between concentric circles of A0 A3
extrude "押し出し3" cut sketch "スケッチ3" against normal through all contours A2
sketch "スケッチ4" plane through (0, 0, 5) normal (0, 0, 1) x (1, 0, 0)
  circle A0 centre (18.9761, 70.4498) radius 8 projected
  circle A1 centre (18.9761, 70.4498) radius 5 projected
  circle A2 centre (18.9761, 70.4498) radius 13.5 projected
  line L0 (18.9761, 86.0901) -> (18.9761, 54.8095)
  line L1 (3.5332, 70.4498) -> (34.419, 70.4498)
  line L2 (17.9761, 83.9127) -> (16.9761, 78.1958)
  line L3 (19.9761, 83.9127) -> (20.9761, 78.1958)
  line L4 (26.7221, 72.4498) -> (32.4391, 71.4498)
  line L5 (26.7221, 68.4498) -> (32.4391, 69.4498)
  circle A3 centre (18.9761, 70.4498) radius 8 projected
  line L6 (20.9761, 62.7038) -> (19.9761, 56.9869)
  line L7 (5.5132, 71.4498) -> (11.2302, 72.4498)
  line L8 (5.5132, 69.4498) -> (11.2302, 68.4498)
  line L9 (16.9761, 62.7038) -> (17.9761, 56.9869)
  point P0 (0, 0)
  dimension "d9" = 1
  dimension "d10" = 1
  dimension "d11" = 1
  dimension "d12" = 1
  dimension "d13" = 1
  dimension "d14" = 1
  dimension "d15" = 1
  dimension "d16" = 1
  dimension "d17" = 2
  dimension "d18" = 2
  dimension "d19" = 2
  dimension "d20" = 2
  dimension "d21" = 2
  dimension "d22" = 2
  dimension "d23" = 2
  dimension "d24" = 2
  constraints: 20 end point, 4 point on circle, 2 midpoint, 1 coincident, 1 horizontal, 1 vertical, 14 other
  measures "d9" distance from line of L0 L2.start
  measures "d10" distance from line of L3.start L0
  measures "d11" distance from line of L1 L4.end
  measures "d12" distance from line of L5.end L1
  measures "d13" distance from line of L0 L6.end
  measures "d14" distance from line of L0 L9.end
  measures "d15" distance from line of L1 L8.start
  measures "d16" distance from line of L1 L7.start
  measures "d17" distance from line of L0 L2.end
  measures "d18" distance from line of L0 L3.end
  measures "d19" distance from line of L1 L4.start
  measures "d20" distance from line of L5.start L1
  measures "d21" distance from line of L0 L6.start
  measures "d22" distance from line of L9.start L0
  measures "d23" distance from line of L1 L8.end
  measures "d24" distance from line of L1 L7.end
extrude "押し出し4" add sketch "スケッチ4" against normal blind 5 contours L1 A2 L5 A0 | A0 L4 A2 L1 | A0 L0 A2 L3 | L6 A2 L0 A0 | A0 L2 A2 L0 | L0 A2 L9 A0 | L1 A2 L7 A0 | A0 L8 A2 L1
fillet "フィレット1" radius 2 16 edges at (5.5132, 71.4498, 2.5) (5.5132, 69.4498, 2.5) (11.2302, 68.4498, 2.5) (11.2302, 72.4498, 2.5) (16.9761, 78.1958, 2.5) (20.9761, 78.1958, 2.5) (17.9761, 83.9127, 2.5) (19.9761, 83.9127, 2.5) (32.4391, 71.4498, 2.5) (32.4391, 69.4498, 2.5) (26.7221, 68.4498, 2.5) (26.7221, 72.4498, 2.5) (20.9761, 62.7038, 2.5) (16.9761, 62.7038, 2.5) (17.9761, 56.9869, 2.5) (19.9761, 56.9869, 2.5)
equation "\"d10\" = d9"
equation "\"d11\" = d10"
equation "\"d12\" = d11"
equation "\"d13\" = d12"
equation "\"d14\" = d13"
equation "\"d15\" = d10"
equation "\"d16\" = d9"
equation "\"d18\" = d17"
equation "\"d19\" = d18"
equation "\"d20\" = d19"
equation "\"d21\" = d20"
equation "\"d22\" = d20"
equation "\"d23\" = d17"
equation "\"d24\" = d23"
